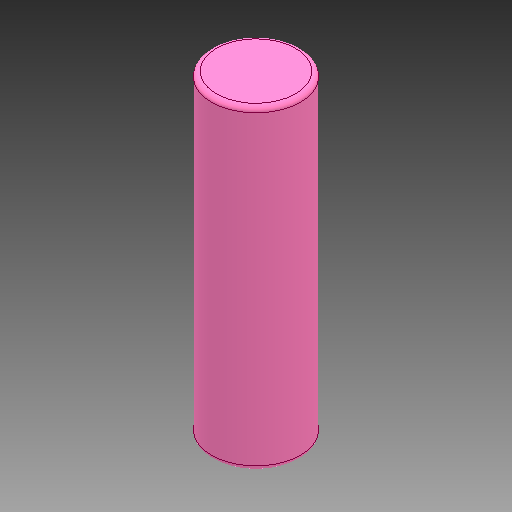
# Autodesk Inventor part: LG INR18650MJ1
Saved by Autodesk Inventor 2018 (Build 220112000, 112)
## iProperties
Created: 2017-08-17
Part Number: LG INR18650MJ1
Material: Kupfer, Guss
Document SubType Name: Modeling
Designer: JochenAlt
Density: 8.94 g/cm^3
Appearance: Pink
Author: JochenAlt
Autodesk Inventor part; units mm, degrees
ref_plane "YZ Plane" through (0, 0, 0) normal (1, 0, 0) x (0, 1, 0)
ref_plane "XZ Plane" through (0, 0, 0) normal (0, 1, 0) x (-1, 0, 0)
ref_plane "XY Plane" through (0, 0, 0) normal (0, 0, 1) x (1, 0, 0)
sketch "Skizze1" plane through (0, 0, 0) normal (0, 0, 1) x (1, 0, 0)
  circle A0 centre (0, 0) radius 9.15
  circle A1 centre (0, 0) radius 4
  dimension "d0" = 18.3
  dimension "d3" = 8
  constraints: 2 centre point, 2 coincident
  measures "d0" diameter of A0
  measures "d3" diameter of A1
extrude "Extrusion1" add sketch "Skizze1" along normal blind 65.1 contours A0 | A1
extrude "Extrusion2" add sketch "Skizze1" against normal blind 1 contours A1
fillet "Rundung1" radius 1 2 edges at (-9.15, 0, 0) (-9.15, 0, 65.1)
